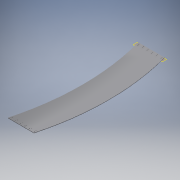
# Autodesk Inventor part: Top_Blade
Saved by Autodesk Inventor 2016 (Build 200138000, 138)
## iProperties
Created: 2016-04-15
Part Number: Top_Blade
Material: Generic
Document SubType Name: Modeling
Designer: 3DPrinterUser
Mass: 2250 g
Surface Area: 9181.77 cm^2
Volume: 2250 cm^3
Density: 1 g/cm^3
Appearance: Default
Author: 3DPrinterUser
Autodesk Inventor part; units mm, degrees
ref_plane "YZ Plane" through (0, 0, 0) normal (1, 0, 0) x (0, 1, 0)
ref_plane "XZ Plane" through (0, 0, 0) normal (0, 1, 0) x (-1, 0, 0)
ref_plane "XY Plane" through (0, 0, 0) normal (0, 0, 1) x (1, 0, 0)
ref_plane "Work Plane1" through (0, 0, 0) normal (0, 0, 1) x (1, 0, 0)
sketch "Sketch1" plane through (0, 0, 0) normal (0, 0, 1) x (1, 0, 0)
  arc A0 (-157.6453, -1471.0012) -> (-157.6453, 28.9988) centre (-2920.1453, -721.0012) ccw projected
  line L0 (142.3547, 28.9988) -> (-157.6453, 28.9988) projected
  arc A1 (142.3547, -1471.0012) -> (142.3547, 28.9988) centre (-2620.1453, -721.0012) ccw projected
  line L1 (142.3547, -1471.0012) -> (-157.6453, -1471.0012) projected
  point P0 (0, 0)
extrude "Extrusion1" add sketch "Sketch1" along normal blind 5
sketch "Sketch2" plane through (0, 0, 5) normal (0, 0, 1) x (1, 0, 0)
  circle A0 centre (-136.8008, 12.9988) radius 3.1 projected
  circle A1 centre (-132.5804, -3.0012) radius 3.1 projected
  circle A2 centre (-83.4222, 12.9988) radius 3.1 projected
  circle A3 centre (-79.2018, -3.0012) radius 3.1 projected
  circle A4 centre (-30.0436, 12.9988) radius 3.1 projected
  circle A5 centre (-25.8232, -3.0012) radius 3.1 projected
  circle A6 centre (23.335, 12.9988) radius 3.1 projected
  circle A7 centre (27.5554, -3.0012) radius 3.1 projected
  circle A8 centre (76.7136, 12.9988) radius 3.1 projected
  circle A9 centre (80.934, -3.0012) radius 3.1 projected
  circle A10 centre (130.0922, 12.9988) radius 3.1 projected
  circle A11 centre (134.3126, -3.0012) radius 3.1 projected
  circle A12 centre (-132.5804, -1439.0012) radius 3.1 projected
  circle A13 centre (-136.8008, -1455.0012) radius 3.1 projected
  circle A14 centre (-79.2018, -1439.0012) radius 3.1 projected
  circle A15 centre (-83.4222, -1455.0012) radius 3.1 projected
  circle A16 centre (-25.8232, -1439.0012) radius 3.1 projected
  circle A17 centre (-30.0436, -1455.0012) radius 3.1 projected
  circle A18 centre (27.5554, -1439.0012) radius 3.1 projected
  circle A19 centre (23.335, -1455.0012) radius 3.1 projected
  circle A20 centre (80.934, -1439.0012) radius 3.1 projected
  circle A21 centre (76.7136, -1455.0012) radius 3.1 projected
  circle A22 centre (134.3126, -1439.0012) radius 3.1 projected
  circle A23 centre (130.0922, -1455.0012) radius 3.1 projected
  point P0 (0, 0)
extrude "Extrusion2" cut sketch "Sketch2" against normal blind 5
body "Solid1"
